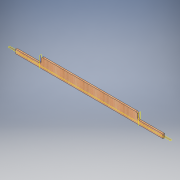
# Autodesk Inventor part: Frame
Saved by Autodesk Inventor 2016 (Build 200138000, 138)
## iProperties
Created: 2015-09-22
Part Number: Frame
Material: Generic
Document SubType Name: Modeling
Designer: xdlea
Density: 1 g/cm^3
Appearance: Birch - Natural Polished
Thickness: 0.750 in
ELength: 12.750 in
Author: xdlea
Autodesk Inventor part; units mm, degrees
ref_plane "YZ Plane" through (0, 0, 0) normal (1, 0, 0) x (0, 1, 0)
ref_plane "XZ Plane" through (0, 0, 0) normal (0, 1, 0) x (-1, 0, 0)
ref_plane "XY Plane" through (0, 0, 0) normal (0, 0, 1) x (1, 0, 0)
sketch "Sketch1" plane through (0, 0, 0) normal (0, 0, 1) x (1, 0, 0)
  line L0 (-609.6, -63.5) -> (609.6, -63.5)
  line L1 (609.6, 63.5) -> (-609.6, 63.5)
  line L2 (-609.6, -63.5) -> (609.6, 63.5) construction
  line L3 (609.6, -63.5) -> (-609.6, 63.5) construction
  line L4 (-609.6, 63.5) -> (-609.6, -12.7)
  line L5 (-609.6, -12.7) -> (-933.45, -12.7)
  line L6 (-933.45, -12.7) -> (-933.45, -63.5)
  line L7 (-933.45, -63.5) -> (-609.6, -63.5)
  line L8 (609.6, -63.5) -> (933.45, -63.5)
  line L9 (933.45, -63.5) -> (933.45, -12.7)
  line L10 (933.45, -12.7) -> (609.6, -12.7)
  line L11 (609.6, -12.7) -> (609.6, 63.5)
  line L12 (0, 88.9) -> (0, -88.9) projected
  point P0 (0, 0)
  dimension "d0" = 127
  dimension "d1" = 1219.2
  dimension "d2" = 323.85
  dimension "d3" = 50.8
  constraints: 24 end point, 4 perpendicular, 4 point on line, 3 symmetric about line, 2 midpoint, 2 vertical, 1 horizontal, 1 parallel, 4 other
  measures "d0" distance between parallel lines of L0 L1
  measures "d1" distance of L1.start L1.end
  measures "d2" distance of L4.end L5.end
  measures "d3" distance between parallel lines of L7 L5
extrude "Extrusion1" add sketch "Sketch1" along normal blind 19.05
fillet "Fillet1" radius 19.05 4 edges at (-609.6, -12.7, 9.525) (-609.6, 63.5, 9.525) (609.6, 63.5, 9.525) (609.6, -12.7, 9.525)
ref_plane "Work Plane2" through (-933.45, -38.1, 19.05) normal (0, 1, 0) x (1, 0, 0)
ref_plane "Work Plane3" through (-628.65, -12.7, 0) normal (-1, 0, 0) x (0, 0, 1)
ref_plane "Work Plane4" through (628.65, -12.7, 0) normal (1, 0, 0) x (0, 0, -1)
equation "\"d2\" = ELength"
equation "\"d3\" = EHeight"
equation "\"d4\" = Thickness"
equation "\"Thickness\" = 19.05"
equation "\"EHeight\" = 50.8"
equation "\"ELength\" = 323.85"
body "Solid1"
